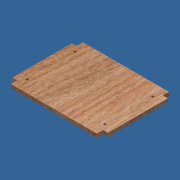
# Autodesk Inventor part: SeitenWand
Saved by Autodesk Inventor 2014 SP2 (Build 180246200, 246)
## iProperties
Created: 2015-02-08
Part Number: SeitenWand
Material: Holz (Birke)
Document SubType Name: Modeling
Designer: 4ndreas
Density: 0.55 g/cm^3
Appearance: Birke - natur - poliert
Author: 4ndreas
Autodesk Inventor part; units mm, degrees
ref_plane "YZ Plane" through (0, 0, 0) normal (1, 0, 0) x (0, 1, 0)
ref_plane "XZ Plane" through (0, 0, 0) normal (0, 1, 0) x (-1, 0, 0)
ref_plane "XY Plane" through (0, 0, 0) normal (0, 0, 1) x (1, 0, 0)
sketch "Skizze1" plane through (0, 0, 0) normal (0, 0, 1) x (1, 0, 0)
  line L0 (-102.3641, 100) -> (-101.6, 100) construction
  line L1 (-101.6, 0) -> (-102.3641, 0) construction
  line L2 (19.2, -16.0826) -> (-120.8, -16.0826) construction
  line L3 (-120.8, -16.0826) -> (-120.8, -13.8079) construction
  line L4 (-120.8, -13.8079) -> (19.2, -13.8079) construction
  line L5 (19.2, -13.8079) -> (19.2, -16.0826) construction
  line L6 (19.2, -28.3315) -> (-120.8, -28.3315) construction
  line L7 (-120.8, -28.3315) -> (-120.8, -24.6314) construction
  line L8 (-120.8, -24.6314) -> (19.2, -24.6314) construction
  line L9 (19.2, -24.6314) -> (19.2, -28.3315) construction
  line L10 (-120.8, 124.6314) -> (-120.8, 128.3315) construction
  line L11 (19.2, 128.3315) -> (19.2, 124.6314) construction
  line L12 (19.2, 116.0826) -> (19.2, 113.8079) construction
  line L13 (0, 100) -> (0.7641, 100) construction
  line L14 (0.7641, 0) -> (0, 0) construction
  line L15 (17.6359, 100) -> (18.4, 100) construction
  line L16 (18.4, 0) -> (17.6359, 0) construction
  line L17 (5.1816, 100) -> (13.2184, 100) construction
  line L18 (13.2184, 0) -> (5.1816, 0) construction
  line L19 (69.2, -3.3397) -> (-120.8, -3.3397) construction
  line L20 (69.2, 103.3397) -> (-120.8, 103.3397) construction
  line L21 (-105.8, 0.0011) -> (54.2, 0.0011)
  line L22 (54.2, 0.0011) -> (54.2, 100.0011)
  line L23 (54.2, 100.0011) -> (-105.8, 100.0011)
  line L24 (-105.8, 100.0011) -> (-105.8, 0.0011)
  line L25 (69.2, -9.3201) -> (-120.8, -9.3201) construction
  line L26 (69.2, 109.0272) -> (-120.8, 109.0272) construction
  line L27 (-100.8, -12.3397) -> (-100.8, 0) construction
  line L28 (49.2, 0) -> (49.2, -12.3397) construction
  line L29 (-100.8, -10.3935) -> (49.2, -10.3935)
  line L30 (49.2, -10.3935) -> (49.2, 110.3935)
  line L31 (49.2, 110.3935) -> (-100.8, 110.3935)
  line L32 (-100.8, 110.3935) -> (-100.8, -10.3935)
  line L33 (-120.8, -7.2256) -> (69.2, -7.2256)
  line L34 (74.2, 45.0011) -> (74.2, -28.46)
  line L35 (74.2, -28.46) -> (69.2, -28.46)
  line L36 (69.2, -28.46) -> (69.2, -6.9656)
  line L37 (69.2, -6.9656) -> (49.2, -6.9656)
  line L38 (49.2, -6.9656) -> (49.2, 0.0011)
  line L39 (49.2, 0.0011) -> (69.2, 0.0011)
  line L40 (69.2, 0.0011) -> (69.2, 45.0011)
  line L41 (69.2, 45.0011) -> (74.2, 45.0011)
  line L42 (69.2, 110.3935) -> (-120.8, 110.3935)
  line L43 (69.2, -11.4055) -> (69.2, -10.3935)
  line L44 (69.2, -10.3935) -> (-120.8, -10.3935)
  dimension "d2" = 5
  dimension "d3" = 5
  dimension "d4" = 100
  constraints: 78 end point, 21 horizontal, 12 vertical, 4 collinear, 4 parallel, 2 perpendicular, 1 point on line, 44 other
  measures "d2" distance between parallel lines of L22 L30
  measures "d3" distance between parallel lines of L32 L24
  measures "d4" distance between parallel lines of L23 L21
extrude "Extrusion1" add sketch "Skizze1" along normal blind 6 contours L30 L23 L22 L21 | L30 L33 L32 L21 | L21 L32 L23 L30 | L21 L24 L23 L32 | L23 L32 L31 L30 | L33 L30 L29 L32
sketch "Skizze2" plane through (0, 0, 6) normal (0, 0, 1) x (1, 0, 0)
  line L0 (49.2, 100.0011) -> (49.2, 110.3935) projected
  line L1 (-100.8, 110.3935) -> (-100.8, 100.0011) projected
  line L2 (-100.8, 100.0011) -> (-105.8, 100.0011) projected
  line L3 (-105.8, 0.0011) -> (-100.8, 0.0011) projected
  line L4 (-100.8, 0.0011) -> (-100.8, -10.3935) projected
  line L5 (49.2, -10.3935) -> (49.2, 0.0011) projected
  line L6 (49.2, 0.0011) -> (54.2, 0.0011) projected
  line L7 (54.2, 100.0011) -> (49.2, 100.0011) projected
  point P0 (0, 0)
  point P1 (39.2, 10.0011)
  point P2 (39.2, 90.0011)
  point P3 (-90.8, 90.0011)
  point P4 (-90.8, 10.0011)
  dimension "d5" = 10
  dimension "d6" = 10
  dimension "d7" = 10
  dimension "d8" = 10
  dimension "d9" = 10
  dimension "d10" = 10
  dimension "d11" = 10
  dimension "d12" = 10
  measures "d5" distance from line of point (-90.8, 10.001) L3
  measures "d6" distance from line of point (-90.8, 10.001) L4
  measures "d7" distance from line of point (-90.8, 90.001) L1
  measures "d8" distance from line of point (-90.8, 90.001) L2
  measures "d9" distance from line of point (39.2, 90.001) L0
  measures "d10" distance from line of point (39.2, 90.001) L7
  measures "d11" distance from line of point (39.2, 10.001) L6
  measures "d12" distance from line of point (39.2, 10.001) L5
hole "Bohrung1" at (39.2, 10.0011, 6) at (39.2, 90.0011, 6) at (-90.8, 90.0011, 6) at (-90.8, 10.0011, 6) direction (0, 0, -1) diameter 4 end through all
sketch "Skizze3" plane through (0, 0, 0) normal (0, 0, -1) x (-1, 0, 0)
  line L0 (105.8, 0.0011) -> (100.8, 0.0011) projected
  line L1 (100.8, 110.3935) -> (100.8, 100.0011) projected
  line L2 (-49.2, 110.3935) -> (100.8, 110.3935) projected
  line L3 (-49.2, 100.0011) -> (-49.2, 110.3935) projected
  line L4 (-49.2, -10.3935) -> (-49.2, 0.0011) projected
  line L5 (100.8, -10.3935) -> (-49.2, -10.3935) projected
  line L6 (100.8, 0.0011) -> (100.8, -10.3935) projected
  line L7 (-49.2, 100.0011) -> (-46.2, 100.0011)
  line L8 (-46.2, 100.0011) -> (-46.2, 110.3935)
  line L9 (-49.2, 0.0011) -> (-46.2, 0.0011)
  line L10 (-46.2, 0.0011) -> (-46.2, -10.3935)
  line L11 (97.8, -10.3935) -> (97.8, 0.0011)
  line L12 (97.8, 0.0011) -> (100.8, 0.0011)
  line L13 (100.8, 100.0011) -> (97.8, 100.0011)
  line L14 (97.8, 100.0011) -> (97.8, 110.3935)
  point P0 (0, 0)
  dimension "d20" = 3
  dimension "d21" = 3
  constraints: 16 end point, 5 perpendicular, 4 point on line, 3 collinear, 2 parallel
  measures "d20" distance between parallel lines of L3 L8
  measures "d21" distance between parallel lines of L14 L1
extrude "Extrusion2" cut sketch "Skizze3" against normal through all
equation "\"d2\" = d3"
equation "\"d7\" = d6"
equation "\"d8\" = d5"
equation "\"d9\" = d8"
equation "\"d10\" = d9"
equation "\"d21\" = d20"
